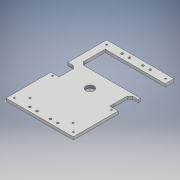
# Autodesk Inventor part: 2枚目
Saved by Autodesk Inventor 2018 (Build 220112000, 112)
## iProperties
Created: 2018-08-15
Part Number: 2枚目
Material: 一般
Document SubType Name: Modeling
Designer: shun2
Density: 1 g/cm^3
Appearance: 既定
Author: shun2
Autodesk Inventor part; units mm, degrees
ref_plane "YZ Plane" through (0, 0, 0) normal (1, 0, 0) x (0, 1, 0)
ref_plane "XZ Plane" through (0, 0, 0) normal (0, 1, 0) x (-1, 0, 0)
ref_plane "XY Plane" through (0, 0, 0) normal (0, 0, 1) x (1, 0, 0)
sketch "スケッチ3" plane through (0, 0, 0) normal (0, 0, 1) x (1, 0, 0)
  line L0 (130, 177.7239) -> (130, 194.7239)
  line L1 (130, 194.7239) -> (0, 194.7239)
  line L2 (0, 0) -> (130, 0)
  line L3 (16, 114.362) -> (16, 86.6)
  line L4 (16, 86.6) -> (0, 86.6)
  circle A0 centre (78, 186.7239) radius 2.15
  circle A1 centre (92, 186.7239) radius 2.15
  circle A2 centre (52, 186.7239) radius 2.15
  circle A3 centre (38, 186.7239) radius 2.15
  circle A4 centre (78, 8) radius 2.15
  circle A5 centre (92, 8) radius 2.15
  circle A6 centre (52, 8) radius 2.15
  circle A7 centre (38, 8) radius 2.15
  line L5 (130, 129.7239) -> (20, 129.7239)
  line L6 (14, 135.7239) -> (14, 177.7239)
  line L7 (14, 177.7239) -> (130, 177.7239)
  line L8 (130, 125.362) -> (119, 125.362)
  line L9 (114, 120.362) -> (114, 86.6)
  line L10 (114, 86.6) -> (130, 86.6)
  line L11 (20, 129.7239) -> (14, 135.7239)
  circle A8 centre (65, 97.362) radius 8
  circle A9 centre (8, 186.7239) radius 1.6
  circle A10 centre (122, 186.7239) radius 1.6
  circle A11 centre (122, 8) radius 1.6
  circle A12 centre (8, 8) radius 1.6
  circle A13 centre (23.2964, 23) radius 1.6
  circle A14 centre (8, 82) radius 1.6
  circle A15 centre (122, 82) radius 1.6
  circle A16 centre (106.7036, 23) radius 1.6
  line L12 (65, 88.362) -> (65, 42.362)
  line L13 (3.4, 186.7239) -> (12.6, 186.7239)
  line L14 (8, 182.1239) -> (8, 191.3239)
  line L15 (117.4, 186.7239) -> (126.6, 186.7239)
  line L16 (122, 182.1239) -> (122, 191.3239)
  line L17 (117.4, 8) -> (126.6, 8)
  line L18 (122, 3.4) -> (122, 12.6)
  line L19 (3.4, 8) -> (12.6, 8)
  line L20 (8, 3.4) -> (8, 12.6)
  line L21 (18.6964, 23) -> (27.8964, 23)
  line L22 (23.2964, 18.4) -> (23.2964, 27.6)
  line L23 (3.4, 82) -> (12.6, 82)
  line L24 (8, 77.4) -> (8, 86.6)
  line L25 (126.6, 82) -> (117.4, 82)
  line L26 (122, 77.4) -> (122, 86.6)
  line L27 (111.3036, 23) -> (102.1036, 23)
  line L28 (106.7036, 18.4) -> (106.7036, 27.6)
  circle A17 centre (92, 186.7239) radius 2.15
  circle A18 centre (78, 186.7239) radius 2.15
  circle A19 centre (52, 186.7239) radius 2.15
  circle A20 centre (38, 186.7239) radius 2.15
  circle A21 centre (65, 97.362) radius 8
  circle A22 centre (92, 8) radius 2.15
  circle A23 centre (78, 8) radius 2.15
  circle A24 centre (52, 8) radius 2.15
  circle A25 centre (38, 8) radius 2.15
  circle A26 centre (23.2964, 23) radius 1.6
  circle A27 centre (8, 8) radius 1.6
  circle A28 centre (122, 8) radius 1.6
  circle A29 centre (106.7036, 23) radius 1.6
  circle A30 centre (122, 82) radius 1.6
  circle A31 centre (122, 186.7239) radius 1.6
  circle A32 centre (8, 186.7239) radius 1.6
  circle A33 centre (8, 82) radius 1.6
  line L29 (0, 0) -> (130, 0)
  line L30 (130, 177.7239) -> (130, 194.7239)
  line L31 (130, 194.7239) -> (0, 194.7239)
  line L32 (130, 177.7239) -> (14, 177.7239)
  line L33 (14, 177.7239) -> (14, 135.7239)
  line L34 (0, 86.6) -> (16, 86.6)
  line L35 (16, 114.362) -> (16, 86.6)
  line L36 (11, 119.362) -> (0, 119.362)
  line L37 (130, 125.362) -> (119, 125.362)
  line L38 (114, 86.6) -> (114, 120.362)
  line L39 (130, 86.6) -> (114, 86.6)
  line L40 (14, 135.7239) -> (20, 129.7239)
  line L41 (0, 194.7239) -> (0, 119.362)
  line L42 (0, 86.6) -> (0, 0)
  line L43 (0, 194.7239) -> (0, 119.362)
  line L44 (0, 86.6) -> (0, 0)
  line L45 (130, 0) -> (130, 86.6)
  line L46 (130, 125.362) -> (130, 129.7239)
  line L47 (130, 0) -> (130, 86.6)
  line L48 (130, 125.362) -> (130, 129.7239)
  line L49 (11, 119.362) -> (16, 114.362)
  line L50 (119, 125.362) -> (114, 120.362)
  point P0 (0, 0)
  point P1 (0, 0)
  constraints: 102 end point, 34 centre point, 17 coincident, 11 collinear, 9 concentric, 4 perpendicular, 2 vertical
sketch "スケッチ4" plane through (0, 0, 0) normal (0, 0, 1) x (1, 0, 0)
  point P0 (0, 0)
extrude "押し出し1" add sketch "スケッチ3" along normal blind 5.5
